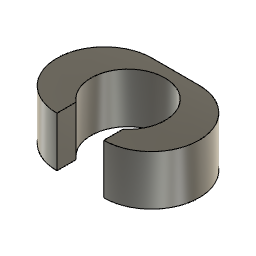
iphone_craddle_connector_fix (Autodesk Fusion 360 design; units mm, degrees)
Autodesk Fusion 360 part; units mm, degrees
sketch "Sketch1" plane through (0, 0, 0) normal (0, 0, 1) x (1, 0, 0)
  line L0 (-0.85, -0.0168) -> (-0.85, 9) construction
  line L1 (6.85, -0.0176) -> (6.85, 9) construction
  line L2 (1.7299, 0) -> (1.7299, 2.58) construction
  line L3 (4.2701, 0) -> (4.2701, 2.58) construction
  line L4 (4.2701, 0) -> (4.2701, -2.58) construction
  line L5 (1.7299, 0) -> (1.7299, -2.58) construction
  line L6 (4.2701, 2.58) -> (1.7299, 2.58)
  line L7 (3, 2.2457) -> (3, -2.58) construction
  arc A0 (1.7299, 2.58) -> (1.7299, -2.58) centre (1.7299, 0) ccw
  arc A1 (4.2701, -2.58) -> (4.2701, 2.58) centre (4.2701, 0) ccw
  line L8 (1.7299, -1.545) -> (1.7299, -2.58)
  line L9 (4.2701, -1.545) -> (4.2701, -2.58)
  arc A2 (4.2701, -1.545) -> (1.7299, -1.545) centre (3, 0) ccw
  dimension "d3" = 7.7
  dimension "d4" = 4
  constraint vertical L0
  constraint vertical L1
  constraint vertical L2
  constraint vertical L3
  constraint parallel L3 L4
  constraint parallel L2 L5
  constraint coincident L7 A2.centre
  constraint coincident L5 L8.start
  constraint coincident L4 L9.start
  measures "d3" distance of L0 L1
  measures "d4" diameter of A2
extrude "Extrude1" add sketch "Sketch1" along normal blind 2.7
